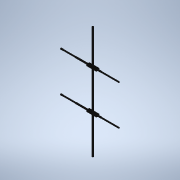
# Autodesk Inventor part: sail_skeleton2
Saved by Autodesk Inventor 2020 (Build 240168000, 168)
## iProperties
Created: 2016-11-10
Part Number: sail_skeleton2
Material: Generic
Document SubType Name: Modeling
Designer: jous
Density: 1 g/cm^3
Appearance: Default
Mass: 887.15 g
Surface Area: 3178.23 cm^2
Volume: 887.15 cm^3
sail_height: 1300.000 mm
tail_offset: 260.000 mm
tail_height: 530.000 mm
Author: jous
Autodesk Inventor part; units mm, degrees
ref_plane "YZ Plane" through (0, 0, 0) normal (1, 0, 0) x (0, 1, 0)
sketch "Sketch1" plane through (0, 0, 0) normal (0, 0, 1) x (1, 0, 0)
  circle A0 centre (0, 0) radius 11
  circle A1 centre (0, 0) radius 9
  dimension "d9" = 22
  dimension "d40" = 18
  constraints: 2 centre point, 2 coincident
  measures "d9" diameter of A0
  measures "d40" diameter of A1
extrude "mast" add sketch "Sketch1" along normal blind 1310 and the other way blind 275
sketch "Sketch4" plane through (0, 0, 0) normal (1, 0, 0) x (0, 1, 0)
  circle A0 centre (0, 818) radius 11
  circle A1 centre (0, 260) radius 11
  line L0 (-20.25, 247.25) -> (20.25, 247.25)
  line L1 (20.25, 247.25) -> (20.25, 272.75)
  line L2 (20.25, 272.75) -> (-20.25, 272.75)
  line L3 (-20.25, 272.75) -> (-20.25, 247.25)
  line L4 (-20.25, 247.25) -> (20.25, 272.75) construction
  line L5 (20.25, 247.25) -> (-20.25, 272.75) construction
  line L6 (-20.25, 805.25) -> (20.25, 805.25)
  line L7 (20.25, 805.25) -> (20.25, 830.75)
  line L8 (20.25, 830.75) -> (-20.25, 830.75)
  line L9 (-20.25, 830.75) -> (-20.25, 805.25)
  line L10 (-20.25, 805.25) -> (20.25, 830.75) construction
  line L11 (20.25, 805.25) -> (-20.25, 830.75) construction
  point P0 (0, 0)
  dimension "d19" = 22
  dimension "d20" = 818
  dimension "d21" = 22
  dimension "d22" = 260
  dimension "d97" = 40.5
  dimension "d98" = 25.5
  dimension "d99" = 40.5
  dimension "d100" = 25.5
  constraints: 24 end point, 4 midpoint, 4 parallel, 2 centre point, 2 horizontal, 2 perpendicular
  measures "d19" diameter of A0
  measures "d20" distance of point (0, 0) A0.centre
  measures "d21" diameter of A1
  measures "d22" distance of point (0, 0) A1.centre
  measures "d97" distance of L2.end L1.end
  measures "d98" distance of L1.end L0.end
  measures "d99" distance of L7.end L8.end
  measures "d100" distance of L6.end L7.end
extrude "tail" add sketch "Sketch4" against normal blind 240 contours A0 | A1
sketch "Sketch8" plane through (-240, 0, 260) normal (-1, 0, 0) x (0, 0, 1)
  circle A0 centre (0, 0) radius 11 projected
  circle A1 centre (0, 0) radius 11
  circle A2 centre (0, 0) radius 9
  circle A3 centre (558, 0) radius 11 projected
  circle A4 centre (558, 0) radius 9
  dimension "d42" = 18
  dimension "d52" = 18
  constraints: 3 centre point, 3 coincident, 1 concentric
  measures "d42" diameter of A2
  measures "d52" diameter of A4
extrude "tail2" add sketch "Sketch8" along normal blind 180 contours A2 | A4
ref_plane "Work Plane4" through (0, 0, 249) normal (0, 0, 1) x (1, 0, 0)
sketch "Sketch11" plane through (-420, 0, 818) normal (-1, 0, 0) x (0, 0, 1)
  circle A0 centre (0, 0) radius 9 projected
  circle A1 centre (-558, 0) radius 11
  circle A2 centre (0, 0) radius 11
  circle A3 centre (0, 0) radius 7
  circle A4 centre (-558, 0) radius 9 projected
  point P0 (-818, 0)
  dimension "d53" = 22
  dimension "d54" = 22
  dimension "d58" = 14
  constraints: 3 centre point, 3 coincident
  measures "d53" diameter of A1
  measures "d54" diameter of A2
  measures "d58" diameter of A3
extrude "tail3" add sketch "Sketch11" along normal blind 30 contours A0 | A1 | A2 | A3 | A4
ref_plane "Work Plane5" through (0, 0, 249) normal (0, 0, 1) x (1, 0, 0)
sketch "Sketch20" plane through (0, 0, 249) normal (0, 0, 1) x (1, 0, 0)
  circle A0 centre (-435, 0) radius 4
  line L0 (-450, 11) -> (-450, -11) projected
  line L1 (-450, 0) -> (-430, 0) construction
  point P0 (0, 0)
  dimension "d82" = 8
  dimension "d83" = 15
  constraints: 2 end point, 1 centre point, 1 midpoint, 1 perpendicular
  measures "d82" diameter of A0
  measures "d83" distance from line of A0.centre L0
extrude "tail holes" cut sketch "Sketch20" along normal through all
sketch "Sketch14" plane through (0, 0, 260) normal (1, 0, 0) x (0, 1, 0)
  circle A0 centre (0, 558) radius 11 projected
  circle A1 centre (0, 0) radius 11 projected
  point P0 (0, -260)
extrude "weight" add sketch "Sketch14" along normal blind 120
sketch "Sketch21" plane through (120, 0, 260) normal (1, 0, 0) x (0, 0, -1)
  circle A0 centre (0, 0) radius 11 projected
  circle A1 centre (0, 0) radius 9
  circle A2 centre (-558, 0) radius 11 projected
  circle A3 centre (-558, 0) radius 9
  point P0 (260, 0)
  dimension "d88" = 18
  dimension "d89" = 18
  constraints: 2 centre point, 2 coincident
  measures "d88" diameter of A1
  measures "d89" diameter of A3
extrude "weight2" add sketch "Sketch21" along normal blind 250 contours A1 | A3
extrude "reinforcement tube" add sketch "Sketch4" along normal mid plane 140
equation "\"tail_height\" = 530"
body "Solid1"
